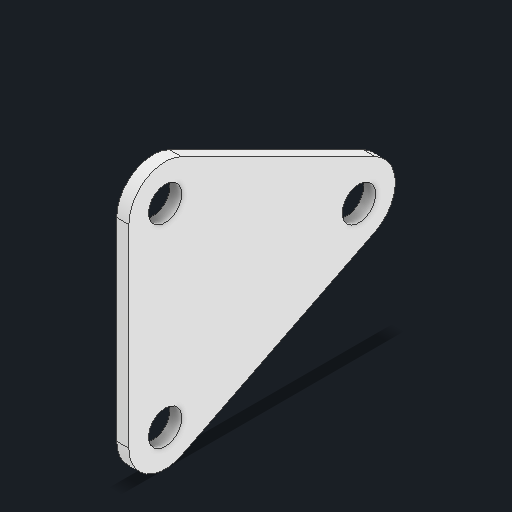
# Autodesk Inventor part: Angle Brace Gusset Bottom
Saved by Autodesk Inventor 2025.1 (Build 291241000, 241)
## iProperties
Created: 2024-12-09
Part Number: Angle Brace Gusset Bottom
Material: Acetal Resin, White
Document SubType Name: Modeling
Designer: avere
Density: 1.425 g/cm^3
Appearance: Smooth - White
Author: avere
Autodesk Inventor part; units mm, degrees
ref_plane "YZ Plane" through (0, 0, 0) normal (1, 0, 0) x (0, 1, 0)
ref_plane "XZ Plane" through (0, 0, 0) normal (0, 1, 0) x (-1, 0, 0)
ref_plane "XY Plane" through (0, 0, 0) normal (0, 0, 1) x (1, 0, 0)
sketch "Sketch1" plane through (0, 0, 0) normal (1, 0, 0) x (0, 1, 0)
  circle A0 centre (18.5414, 11.8362) radius 2.1844
  circle A1 centre (-6.8586, 11.8362) radius 2.1844
  arc A2 (22.8019, 9.708) -> (18.5414, 16.5987) centre (18.5414, 11.8362) ccw
  arc A3 (-6.8586, 16.5987) -> (-11.1175, 9.7048) centre (-6.8586, 11.8362) ccw
  arc A4 (1.5942, -15.6954) -> (10.1136, -15.6922) centre (5.8531, -13.564) ccw
  circle A5 centre (5.8528, -13.5638) radius 2.1971
  line L0 (18.5414, 16.5987) -> (-6.8586, 16.5987)
  line L1 (22.8019, 9.708) -> (10.1136, -15.6922)
  line L2 (-11.1175, 9.7048) -> (1.5942, -15.6954)
  point P0 (0, 0)
  dimension "d0" = 9.525
  dimension "d1" = 9.525
  dimension "d2" = 9.525
  constraints: 6 centre point, 6 end point, 6 point on circle, 4 tangent, 2 coincident, 1 horizontal
  measures "d0" diameter of A2
  measures "d1" diameter of A3
  measures "d2" diameter of A4
extrude "Extrusion1" add sketch "Sketch1" along normal blind 1.5875
body "Solid1"
